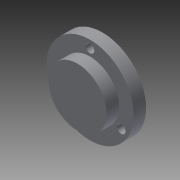
# Autodesk Inventor part: 7.1 Part 6
Saved by Autodesk Inventor 2015 (Build 190159000, 159)
## iProperties
Created: 2015-03-06
Part Number: 7.1 Part 6
Material: Generic
Document SubType Name: Modeling
Designer: PLTW-Stu-02
Density: 1 g/cm^3
Appearance: Default
Author: PLTW-Stu-02
Autodesk Inventor part; units mm, degrees
ref_plane "YZ Plane" through (0, 0, 0) normal (1, 0, 0) x (0, 1, 0)
ref_plane "XZ Plane" through (0, 0, 0) normal (0, 1, 0) x (-1, 0, 0)
ref_plane "XY Plane" through (0, 0, 0) normal (0, 0, 1) x (1, 0, 0)
sketch "Sketch1" plane through (0, 0, 0) normal (0, 0, 1) x (1, 0, 0)
  circle A0 centre (27.3374, 23.6131) radius 22.225
  point P0 (0, 0)
  dimension "d0" = 44.45
  constraints: 1 centre point
  measures "d0" diameter of A0
extrude "Extrusion1" add sketch "Sketch1" along normal blind 6.35
sketch "Sketch2" plane through (27.3374, 23.6131, 6.35) normal (0, 0, 1) x (1, 0, 0)
  circle A0 centre (0, 0) radius 14.7955
  point P0 (-27.3374, -23.6131)
  dimension "d3" = 29.591
  constraints: 1 centre point
  measures "d3" diameter of A0
extrude "Extrusion2" add sketch "Sketch2" along normal blind 6.35
sketch "Sketch4" plane through (27.3374, 23.6131, 0) normal (0, 0, -1) x (-1, 0, 0)
  circle A0 centre (0, 0) radius 18.415
  circle A1 centre (0, 18.415) radius 2.1844
  circle A2 centre (15.9479, -9.2075) radius 2.1844
  circle A3 centre (-15.9479, -9.2075) radius 2.1844
  point P0 (27.3374, -23.6131)
  dimension "d14" = 360
  constraints: 4 coincident, 3 centre point, 1 vertical alignment, 9 other
hole "Hole1" at (27.3374, 42.0281, 0) at (43.2853, 14.4056, 0) at (11.3896, 14.4056, 0) direction (0, 0, 1) diameter 4.3688 depth 25.4 tip angle 118
body "Solid1"
